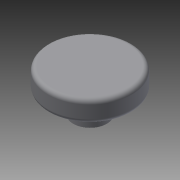
# Autodesk Inventor part: Fixture_Knob_1
Saved by Autodesk Inventor 2015 (Build 190159000, 159)
## iProperties
Created: 2014-12-16
Part Number: Fixture_Knob_1
Material: Generic
Document SubType Name: Modeling
Designer: amarschn
Density: 1 g/cm^3
Appearance: Default
Author: amarschn
Autodesk Inventor part; units mm, degrees
ref_plane "YZ Plane" through (0, 0, 0) normal (1, 0, 0) x (0, 1, 0)
ref_plane "XZ Plane" through (0, 0, 0) normal (0, 1, 0) x (-1, 0, 0)
ref_plane "XY Plane" through (0, 0, 0) normal (0, 0, 1) x (1, 0, 0)
sketch "Sketch1" plane through (0, 0, 0) normal (1, 0, 0) x (0, 1, 0)
  line L0 (0, 0) -> (0, -22.86)
  line L1 (-2.54, -25.4) -> (-10.16, -25.4)
  line L2 (-12.7, -22.86) -> (-12.7, -10.16)
  line L3 (-12.7, -10.16) -> (-25.4, -10.16)
  line L4 (-25.4, -10.16) -> (-25.4, 0)
  line L5 (-25.4, 0) -> (0, 0)
  arc A0 (-2.54, -25.4) -> (0, -22.86) centre (-2.54, -22.86) ccw
  arc A1 (-12.7, -22.86) -> (-10.16, -25.4) centre (-10.16, -22.86) ccw
  point P0 (0, -25.4)
  point P1 (-12.7, -25.4)
  dimension "d0" = 25.4
  dimension "d1" = 10.16
  dimension "d2" = 12.7
  dimension "d3" = 25.4
  dimension "d4" = 2.54
  constraints: 12 end point, 5 perpendicular, 4 point on circle, 4 point on line, 4 tangent, 2 centre point, 1 equal radius, 1 vertical
  measures "d0" distance of L0.start point (0, -25.4)
  measures "d1" distance of L3.end L4.end
  measures "d2" distance of point (0, -25.4) point (-12.7, -25.4)
  measures "d3" distance of L4.end L0.start
  measures "d4" radius of A0
revolve "Revolution1" add sketch "Sketch1" angle 360 about axis through (0, -25.4, 0) along (0, 1, 0)
body "Solid1"
